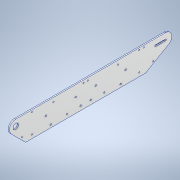
# Autodesk Inventor part: plyta_glowna_V3
Saved by Autodesk Inventor 2020.3 (Build 243373000, 373)
## iProperties
Created: 2021-04-10
Part Number: plyta_glowna_V3
Material: Aluminium 6061
Document SubType Name: Modeling
Designer: patryk.szydlik
Density: 2.7 g/cm^3
Appearance: Aluminium — płaski
Mass: 531.743 g
Surface Area: 1004.37 cm^2
Volume: 196.942 cm^3
Author: patryk.szydlik
Autodesk Inventor part; units mm, degrees
ref_plane "YZ Plane" through (0, 0, 0) normal (1, 0, 0) x (0, 1, 0)
ref_plane "XZ Plane" through (0, 0, 0) normal (0, 1, 0) x (-1, 0, 0)
ref_plane "XY Plane" through (0, 0, 0) normal (0, 0, 1) x (1, 0, 0)
sketch "Sketch2" plane through (0, 0, 0) normal (1, 0, 0) x (0, 1, 0)
  line L0 (127.2876, 96.9132) -> (-12.7124, 96.9132) construction
  line L1 (-12.7124, 96.9132) -> (-12.7124, -363.0868) construction
  line L2 (-12.7124, -363.0868) -> (127.2876, -363.0868) construction
  line L3 (127.2876, -363.0868) -> (127.2876, 96.9132) construction
  line L4 (97.2876, 66.9132) -> (17.2876, 66.9132) construction
  line L5 (17.2876, 66.9132) -> (17.2876, -333.0868) construction
  line L6 (17.2876, -333.0868) -> (97.2876, -333.0868) construction
  line L7 (97.2876, -333.0868) -> (97.2876, 66.9132) construction
  point P0 (0, 0)
  dimension "d2" = 140
  dimension "d3" = 460
  dimension "d4" = 80
  dimension "d5" = 400
  dimension "d6" = 30
  dimension "d7" = 30
  constraints: 16 end point, 4 parallel, 2 horizontal, 2 perpendicular
  measures "d2" distance of L2.end L1.end
  measures "d3" distance of L1.end L0.end
  measures "d4" distance of L6.end L5.end
  measures "d5" distance of L5.end L4.end
  measures "d6" distance between parallel lines of L3 L7
  measures "d7" distance between parallel lines of L0 L4
sketch "Sketch3" plane through (0, 0, 0) normal (1, 0, 0) x (0, 1, 0)
  circle A0 centre (-62.7124, 66.9132) radius 20
  line L0 (-12.7124, 96.9132) -> (-12.7124, -363.0868) construction
  circle A1 centre (-62.7124, -13.0868) radius 20
  circle A2 centre (-62.7124, -93.0868) radius 20
  circle A3 centre (-62.7124, -173.0868) radius 20
  circle A4 centre (-62.7124, -253.0868) radius 20
  circle A5 centre (-62.7124, -333.0868) radius 20
  line L1 (127.2876, 96.9132) -> (-12.7124, 96.9132) construction
  point P0 (0, 0)
  dimension "d8" = 40
  dimension "d9" = 50
  dimension "d12" = 80
  dimension "d17" = 30
  constraints: 6 centre point, 1 vertical, 10 other
  measures "d8" diameter of A0
  measures "d9" distance from line of L0 A0.centre
  measures "d12" distance of A0.centre A1.centre
  measures "d17" distance from line of A0.centre L1
sketch "Sketch1" plane through (0, 0, 0) normal (1, 0, 0) x (0, 1, 0)
  circle A0 centre (45.5719, 146.9132) radius 40
  circle A1 centre (85.5719, -453.0868) radius 40
  line L0 (127.2876, 96.9132) -> (-12.7124, 96.9132) construction
  line L1 (-12.7124, -363.0868) -> (127.2876, -363.0868) construction
  line L2 (-62.7124, 66.9132) -> (-62.7124, -13.0868) construction
  line L3 (-62.7124, -253.0868) -> (-62.7124, -333.0868) construction
  line L4 (85.2399, 141.7706) -> (125.4799, -450.3748) construction
  circle A2 centre (-62.7124, 66.9132) radius 20 projected
  line L5 (17.2876, 175.1975) -> (-76.8545, 81.0553)
  circle A3 centre (-62.7124, -333.0868) radius 20 projected
  line L6 (-76.8545, -347.2289) -> (57.2876, -481.3711) construction
  point P0 (0, 0)
  dimension "d0" = 80
  dimension "d1" = 80
  dimension "d18" = 50
  dimension "d19" = 90
  dimension "d45" = 135
  dimension "d46" = 135
  constraints: 10 end point, 4 point on circle, 3 tangent, 2 centre point, 2 coincident, 2 vertical, 6 other
  measures "d0" diameter of A0
  measures "d1" diameter of A1
  measures "d18" distance from line of A0.centre L0
  measures "d19" distance from line of A1.centre L1
  measures "d45" angle of L2 L5
  measures "d46" angle of L3 L6
sketch "Sketch4" plane through (0, 0, 0) normal (1, 0, 0) x (0, 1, 0)
  line L0 (37.6815, -3.0868) -> (-57.7124, 26.9132) construction
  circle A0 centre (-62.7124, 66.9132) radius 20 projected
  circle A1 centre (-62.7124, -13.0868) radius 20 projected
  line L1 (-62.7124, 66.9132) -> (-62.7124, -13.0868) construction
  circle A2 centre (-27.7124, 112.5679) radius 20 construction
  circle A3 centre (-27.7124, 32.5679) radius 20 construction
  line L2 (-27.7124, 72.5679) -> (37.6815, -3.0868) construction
  line L3 (-27.7124, 72.5679) -> (-57.7124, 26.9132) construction
  line L4 (37.6815, -3.0868) -> (-42.7124, 49.7406) construction
  line L5 (-12.7124, 96.9132) -> (-12.7124, -363.0868) construction
  point P0 (0, 0)
  point P1 (-61.7124, 47.9132)
  point P2 (83.0715, 79.9132)
  point P3 (83.0715, -80.0868)
  point P4 (37.6815, -163.0868)
  point P5 (83.0715, -240.0868)
  point P6 (37.6815, -323.0868)
  dimension "d22" = 40
  dimension "d23" = 5
  dimension "d24" = 30
  dimension "d25" = 40
  dimension "d26" = 40
  dimension "d27" = 80
  dimension "d28" = 40
  dimension "d29" = 100
  dimension "d30" = 100
  dimension "d31" = 35
  dimension "d32" = 54.6292
  dimension "d33" = 27.3146
  dimension "d34" = 56.691
  dimension "d35" = 95.3939
  dimension "d36" = 45.39
  dimension "d37" = 83
  dimension "d40" = 160
  constraints: 8 end point, 2 centre point, 2 vertical alignment, 1 coincident, 1 midpoint, 1 vertical, 4 other
  measures "d22" vertical distance of point (-62.712, 66.913) L0.end
  measures "d23" horizontal distance of point (-62.712, 66.913) L0.end
  measures "d24" vertical distance of L0.end L0.start
  measures "d25" diameter of A3
  measures "d26" diameter of A2
  measures "d27" distance of A3.centre A2.centre
  measures "d28" distance of A3.centre L2.start
  measures "d29" distance of L0.start L0.end
  measures "d30" distance of L2.start L0.start
  measures "d31" horizontal distance of point (-62.712, 66.913) A2.centre
  measures "d32" distance of L0.end L2.start
  measures "d33" distance of L0.end L4.end
  measures "d34" angle of L5 L4
  measures "d35" horizontal distance of L0.end L0.start
  measures "d36" horizontal distance of L0.start point (83.072, 79.913)
  measures "d37" vertical distance of L0.start point (83.072, 79.913)
  measures "d40" distance of point (83.072, 79.913) point (83.072, -80.087)
sketch "Sketch6" plane through (0, 0, 0) normal (1, 0, 0) x (0, 1, 0)
  line L0 (234.6261, -208.0868) -> (-157.479, -208.0868) construction
  line L1 (237.7494, -58.0868) -> (-154.3557, -58.0868) construction
  line L2 (17.2876, -333.0868) -> (97.2876, -333.0868) construction
  line L3 (97.2876, 66.9132) -> (17.2876, 66.9132) construction
  point P0 (0, 0)
  dimension "d61" = 125
  dimension "d62" = 125
  constraints: 4 end point, 2 horizontal
  measures "d61" distance between parallel lines of L1 L3
  measures "d62" distance between parallel lines of L2 L0
sketch "Sketch5" plane through (0, 0, 0) normal (1, 0, 0) x (0, 1, 0)
  arc A0 (90.5716, 146.9132) -> (47.894, 164.5909) centre (65.5716, 146.9132) ccw
  arc A1 (90.5716, -453.0868) -> (43.921, -465.5868) centre (65.5716, -453.0868) ccw construction
  line L0 (90.5716, -453.0868) -> (90.5716, 146.9132)
  arc A2 (47.894, 164.5909) -> (90.5716, 146.9132) centre (65.5716, 146.9132) ccw construction
  arc A3 (43.921, -465.5868) -> (90.5716, -453.0868) centre (65.5716, -453.0868) ccw
  arc A4 (62.5716, -453.0868) -> (68.5716, -453.0868) centre (65.5716, -453.0868) ccw
  arc A5 (68.5716, -413.0868) -> (62.5716, -413.0868) centre (65.5716, -413.0868) ccw
  line L1 (68.5716, -413.0868) -> (68.5716, -453.0868)
  line L2 (62.5716, -413.0868) -> (62.5716, -453.0868)
  arc A6 (68.5716, -453.0868) -> (62.5716, -453.0868) centre (65.5716, -453.0868) ccw construction
  arc A7 (62.5716, -413.0868) -> (68.5716, -413.0868) centre (65.5716, -413.0868) ccw construction
  line L3 (114.7874, 96.9132) -> (-25.2126, 96.9132) construction
  line L4 (-32.7126, -363.0868) -> (107.2874, -363.0868) construction
  line L5 (217.7491, -58.0868) -> (-174.356, -58.0868) construction
  line L6 (214.6258, -208.0868) -> (-177.4793, -208.0868) construction
  circle A8 centre (65.5716, 146.9132) radius 11
  circle A9 centre (65.5716, -413.0868) radius 50 construction
  circle A10 centre (65.5716, 146.9132) radius 55 construction
  line L7 (-9.4284, 107.2685) -> (47.894, 164.5909)
  line L8 (43.921, -465.5868) -> (-9.4284, -373.183)
  line L9 (-9.4284, -373.183) -> (-9.4284, 107.2685)
  line L10 (-2.7126, 66.9132) -> (-2.7126, -333.0868) construction
  line L11 (-62.7124, -13.0868) -> (-62.7124, -93.0868) construction
  line L12 (-62.7124, -173.0868) -> (-62.7124, -253.0868) construction
  point P0 (0, 0)
  point P1 (83.0716, 81.9132)
  point P2 (83.0716, -348.0868)
  point P3 (83.0716, -366.2493)
  point P4 (16.3276, 122.4179)
  point P5 (5.5716, -347.5476)
  point P6 (16.5597, -403.1957)
  point P7 (8.0719, -82.4742)
  point P8 (8.0719, -243.0868)
  point P9 (-17.7126, -58.0868)
  point P10 (-17.7126, -208.0868)
  point P11 (5.5716, 81.9132)
  point P12 (-62.7124, 66.9132)
  point P13 (-62.7124, -333.0868)
  point P14 (-62.7124, -53.0868)
  point P15 (-62.7124, -213.0868)
  point P16 (2.2876, 6.9132)
  point P17 (42.2876, 26.9132)
  point P18 (47.2876, -93.0868)
  point P19 (7.2876, -113.0868)
  point P20 (7.2876, -153.0868)
  point P21 (47.2876, -173.0868)
  point P22 (42.2876, -293.0868)
  point P23 (2.2876, -273.0868)
  point P24 (2.2876, 6.9132)
  point P25 (-62.7124, 66.9132)
  point P26 (5.5716, -208.0868)
  point P27 (5.5716, -58.0868)
  point P28 (75.1946, -4.4068)
  point P29 (80.1946, -124.4068)
  point P30 (80.1946, -141.7668)
  point P31 (75.1946, -261.7668)
  dimension "d84" = 110
  dimension "d47" = 50
  dimension "d48" = 50
  dimension "d58" = 6
  dimension "d59" = 6
  dimension "d60" = 40
  dimension "d63" = 15
  dimension "d64" = 7.5
  dimension "d65" = 15
  dimension "d66" = 7.5
  dimension "d81" = 22
  dimension "d82" = 100
  dimension "d86" = 100
  dimension "d92" = 7.5
  dimension "d101" = 7.5
  dimension "d102" = 7.5
  dimension "d103" = 135
  dimension "d104" = 150
  dimension "d151" = 15
  dimension "d155" = 15
  dimension "d159" = 15
  dimension "d160" = 15
  dimension "d163" = 60
  dimension "d164" = 65
  dimension "d165" = 20
  dimension "d166" = 40
  dimension "d174" = 60
  dimension "d175" = 70
  dimension "d176" = 40
  dimension "d177" = 20
  dimension "d196" = 128.284
  dimension "d197" = 15
  dimension "d198" = 11.32
  dimension "d199" = 72.907
  dimension "d200" = 11.32
  dimension "d201" = 72.907
  dimension "d204" = 11.32
  dimension "d213" = 65
  dimension "d214" = 40
  dimension "d215" = 20
  dimension "d216" = 20
  dimension "d217" = 40
  constraints: 26 end point, 18 point on circle, 10 centre point, 8 coincident, 4 point on line, 2 midpoint, 1 vertical alignment, 3 other
  measures "d47" diameter of A0
  measures "d48" diameter of A1
  measures "d58" diameter of A4
  measures "d59" diameter of A5
  measures "d60" distance of point (65.572, -453.087) point (65.572, -413.087)
  measures "d63" distance from line of L3 point (83.072, 81.913)
  measures "d64" distance from line of L0 point (83.072, 81.913)
  measures "d65" distance from line of L4 point (83.072, -348.087)
  measures "d66" distance from line of L0 point (83.072, -348.087)
  measures "d81" diameter of A8
  measures "d82" diameter of A9
  measures "d86" distance between parallel lines of L9 L0
  measures "d92" distance from line of L0 A9.start
  measures "d101" distance from line of point (16.328, 122.418) L7
  measures "d102" distance from line of L8 A9.end
  measures "d103" angle of L7 L9
  measures "d104" angle of L9 L8
  measures "d151" distance from line of L10 point (-17.713, -58.087)
  measures "d155" distance from line of L10 point (-17.713, -208.087)
  measures "d159" distance from line of L3 point (5.572, 81.913)
  measures "d160" distance from line of L9 point (5.572, 81.913)
  measures "d163" vertical distance of point (-62.712, 66.913) point (2.288, 6.913)
  measures "d164" horizontal distance of point (-62.712, 66.913) point (2.288, 6.913)
  measures "d165" vertical distance of point (2.288, 6.913) point (42.288, 26.913)
  measures "d166" horizontal distance of point (2.288, 6.913) point (42.288, 26.913)
  measures "d174" vertical distance of point (-62.712, -213.087) point (7.288, -153.087)
  measures "d175" horizontal distance of point (-62.712, -213.087) point (7.288, -153.087)
  measures "d176" horizontal distance of point (47.288, -173.087) point (7.288, -153.087)
  measures "d177" vertical distance of point (47.288, -173.087) point (7.288, -153.087)
  measures "d196" horizontal distance of point (65.572, 146.913) point (-62.712, 66.913)
  measures "d197" distance from line of point (5.572, -347.548) L9
  measures "d198" vertical distance of point (75.195, -4.407) point (2.288, 6.913)
  measures "d199" horizontal distance of point (2.288, 6.913) point (75.195, -4.407)
  measures "d200" vertical distance of point (7.288, -113.087) point (80.195, -124.407)
  measures "d201" horizontal distance of point (7.288, -113.087) point (80.195, -124.407)
  measures "d204" vertical distance of point (2.288, -273.087) point (75.195, -261.767)
  measures "d213" horizontal distance of point (2.288, -273.087) L12.end
  measures "d214" horizontal distance of point (2.288, -273.087) point (42.288, -293.087)
  measures "d215" vertical distance of point (2.288, -273.087) point (42.288, -293.087)
  measures "d216" vertical distance of point (7.288, -113.087) point (47.288, -93.087)
  measures "d217" horizontal distance of point (47.288, -93.087) point (7.288, -113.087)
extrude "Extrusion1" add sketch "Sketch5" against normal blind 5
hole "Hole1" at (0, 83.0716, 81.9132) at (0, 16.3276, 122.4179) at (0, 5.5716, -347.5476) at (0, 16.5597, -403.1957) at (0, 83.0716, -348.0868) at (0, 83.0716, -366.2493) at (0, -17.7126, -58.0868) at (0, -17.7126, -208.0868) at (0, 5.5716, 81.9132) at (0, 5.5716, -58.0868) at (0, 5.5716, -208.0868) direction (-1, 0, 0) diameter 5 end through all clearance for "Flat Head Machine Screw" size "M5" standard "Ansi Metric M Profile"
sketch "Sketch7" plane through (0, 0, 0) normal (1, 0, 0) x (0, 0, -1)
  circle A0 centre (348.0868, 83.0716) radius 2.5 projected
  circle A1 centre (-122.4179, 16.3276) radius 2.5 projected
  circle A2 centre (-81.9132, 83.0716) radius 2.5 projected
  circle A3 centre (403.1957, 16.5597) radius 2.5 projected
  circle A4 centre (366.2493, 83.0716) radius 2.5 projected
  line L0 (373.183, -9.4284) -> (465.5868, 43.921) projected
  arc A5 (465.5868, 43.921) -> (453.0868, 90.5716) centre (453.0868, 65.5716) ccw projected
  line L1 (453.0868, 90.5716) -> (-146.9132, 90.5716) projected
  arc A6 (-146.9132, 90.5716) -> (-164.5909, 47.894) centre (-146.9132, 65.5716) ccw projected
  line L2 (-164.5909, 47.894) -> (-107.2685, -9.4284) projected
  circle A7 centre (-146.9132, 65.5716) radius 11 projected
  arc A8 (453.0868, 62.5716) -> (453.0868, 68.5716) centre (453.0868, 65.5716) ccw projected
  line L3 (453.0868, 62.5716) -> (413.0868, 62.5716) projected
  arc A9 (413.0868, 68.5716) -> (413.0868, 62.5716) centre (413.0868, 65.5716) ccw projected
  line L4 (413.0868, 68.5716) -> (453.0868, 68.5716) projected
  line L5 (-146.9132, 75.5716) -> (453.0868, 75.5716)
  arc A10 (458.0868, 56.9114) -> (453.0868, 75.5716) centre (453.0868, 65.5716) ccw
  line L6 (458.0868, 56.9114) -> (386.4847, 15.5719)
  line L7 (386.4847, 15.5719) -> (398.0868, 15.5719)
  line L8 (-111.0556, 15.5719) -> (-153.9843, 58.5006)
  arc A11 (-146.9132, 75.5716) -> (-153.9843, 58.5006) centre (-146.9132, 65.5716) ccw
  line L9 (453.0868, 90.5716) -> (-146.9132, 90.5716) projected
  line L10 (-91.9132, 90.5716) -> (-71.9132, 90.5716)
  line L11 (-71.9132, 90.5716) -> (-71.9132, 0.5716)
  line L12 (-71.9132, 0.5716) -> (-91.9132, 0.5716)
  line L13 (-91.9132, 0.5716) -> (-91.9132, 90.5716)
  line L14 (-107.2685, -9.4284) -> (373.183, -9.4284) projected
  line L15 (48.0868, 90.5716) -> (68.0868, 90.5716)
  line L16 (68.0868, 90.5716) -> (68.0868, -9.4284)
  line L17 (68.0868, -9.4284) -> (48.0868, -9.4284)
  line L18 (48.0868, -9.4284) -> (48.0868, 90.5716)
  line L19 (198.0868, 90.5716) -> (218.0868, 90.5716)
  line L20 (218.0868, 90.5716) -> (218.0868, -9.4284)
  line L21 (218.0868, -9.4284) -> (198.0868, -9.4284)
  line L22 (198.0868, -9.4284) -> (198.0868, 90.5716)
  line L23 (338.0868, 90.5716) -> (358.0868, 90.5716)
  line L24 (358.0868, 90.5716) -> (358.0868, 38.7433)
  line L25 (358.0868, -9.4284) -> (338.0868, -9.4284)
  line L26 (338.0868, -9.4284) -> (338.0868, 90.5716)
  circle A12 centre (-146.9132, 65.5719) radius 25 construction
  arc A13 (453.0868, 62.5716) -> (453.0868, 68.5716) centre (453.0868, 65.5716) ccw construction
  circle A14 centre (453.0868, 65.5716) radius 25 construction
  arc A15 (413.0868, 68.5716) -> (413.0868, 62.5716) centre (413.0868, 65.5716) ccw construction
  line L27 (-146.9132, 90.5716) -> (453.0868, 90.5716) construction
  line L28 (398.0911, 65.9311) -> (398.0911, 90.5716) construction
  line L29 (403.0868, 38.7433) -> (456.6188, 38.7433) construction
  line L30 (465.5868, 43.921) -> (373.183, -9.4284) construction
  line L31 (403.0868, 38.7433) -> (403.0868, 15.5719) construction
  line L32 (398.0868, 65.5716) -> (398.0868, 38.7433) construction
  line L33 (398.0868, 38.7433) -> (398.0868, 38.7433) construction
  line L34 (398.0868, 15.5719) -> (398.0868, 38.7433) construction
  line L35 (408.0868, 38.7433) -> (408.0868, 15.5716) construction
  line L36 (358.0868, 38.7433) -> (358.0868, -9.4284)
  line L37 (398.0868, 38.7433) -> (403.0868, 38.7433) construction
  line L38 (398.0868, 15.5719) -> (-111.0556, 15.5719)
  line L39 (218.0868, 75.5716) -> (338.0868, 15.5719) construction
  line L40 (218.0868, 15.5719) -> (338.0868, 75.5716) construction
  line L41 (326.9064, 75.5716) -> (218.0868, 21.1621) construction
  line L42 (229.2672, 15.5719) -> (338.0868, 69.9815) construction
  line L43 (229.2672, 75.5716) -> (338.0868, 21.1621) construction
  line L44 (218.0868, 69.9815) -> (326.9064, 15.5719) construction
  line L45 (333.0869, 67.4815) -> (333.0869, 23.662) construction
  line L46 (68.0868, 75.5716) -> (198.0868, 15.5719) construction
  line L47 (198.0868, 75.5716) -> (68.0868, 15.5719) construction
  line L48 (68.0868, 21.0787) -> (186.1552, 75.5716) construction
  line L49 (80.0184, 15.5719) -> (198.0868, 70.0648) construction
  line L50 (198.0868, 21.0787) -> (80.0184, 75.5716) construction
  line L51 (68.0868, 70.0648) -> (186.1552, 15.5719) construction
  line L52 (48.0868, 15.5719) -> (-71.9132, 75.5716) construction
  line L53 (-71.9132, 15.5719) -> (48.0868, 75.5716) construction
  line L54 (36.9064, 75.5716) -> (-71.9132, 21.1621) construction
  line L55 (-60.7328, 15.5719) -> (48.0868, 69.9815) construction
  line L56 (-60.7328, 75.5716) -> (48.0868, 21.1621) construction
  line L57 (-71.9132, 69.9815) -> (36.9064, 15.5719) construction
  line L58 (68.0868, 73.0713) -> (61.5727, 73.0713) construction
  line L59 (48.0868, 47.6814) -> (-4.9521, 47.6814) construction
  line L60 (198.0868, 47.6814) -> (140.4475, 47.6814) construction
  line L61 (218.0868, 73.0713) -> (211.9072, 73.0713) construction
  line L62 (-121.9132, 65.5719) -> (-121.9132, 75.5716) construction
  line L63 (-121.9132, 65.5719) -> (-121.9132, 26.4295) construction
  line L64 (-121.9132, 75.5716) -> (-91.9132, 15.5719) construction
  line L65 (-91.9132, 26.7522) -> (-116.323, 75.5716) construction
  line L66 (-121.9132, 64.3913) -> (-97.5034, 15.5719) construction
  line L67 (-111.0556, 15.5719) -> (-121.9132, 15.5719) construction
  line L68 (-121.9132, 15.5719) -> (-121.9132, 26.4295) construction
  line L69 (-121.9132, 15.5719) -> (-91.9132, 75.5716) construction
  line L70 (-97.5034, 75.5716) -> (-121.9132, 26.7522) construction
  line L71 (-116.323, 15.5719) -> (-91.9132, 64.3913) construction
  circle A16 centre (413.0868, 65.5716) radius 15 construction
  line L72 (398.0911, 75.5716) -> (358.0868, 15.5719) construction
  line L73 (398.0868, 15.5719) -> (358.0868, 75.5716) construction
  line L74 (392.0816, 75.5716) -> (358.0868, 24.5851) construction
  line L75 (398.0911, 66.5584) -> (364.0963, 15.5719) construction
  line L76 (358.0868, 66.5578) -> (392.0775, 15.5719) construction
  line L77 (398.0868, 24.5857) -> (364.0961, 75.5716) construction
  line L78 (-107.2685, -9.4284) -> (373.183, -9.4284) projected
  point P0 (0, 0)
  dimension "d93" = 15
  dimension "d94" = 10
  dimension "d95" = 20
  dimension "d97" = 20
  dimension "d99" = 20
  dimension "d100" = 10
  dimension "d105" = 20
  dimension "d107" = 5
  dimension "d108" = 5
  dimension "d111" = 5
  dimension "d112" = 5
  dimension "d113" = 5
  dimension "d114" = 5
  dimension "d116" = 5
  dimension "d117" = 5
  dimension "d118" = 5
  dimension "d119" = 5
  dimension "d120" = 5
  dimension "d121" = 5
  dimension "d122" = 5
  dimension "d123" = 5
  dimension "d128" = 5
  dimension "d129" = 5
  dimension "d130" = 5
  dimension "d131" = 5
  dimension "d132" = 30
  dimension "d133" = 5
  dimension "d134" = 5
  dimension "d135" = 5
  dimension "d136" = 5
  constraints: 134 end point, 57 point on line, 29 parallel, 11 perpendicular, 9 horizontal, 6 point on circle, 6 vertical, 4 centre point, 3 coincident, 1 collinear, 1 concentric, 1 horizontal alignment, 1 vertical alignment, 54 other
  measures "d94" distance from line of L11 A2.centre
  measures "d95" distance of L16.end L17.end
  measures "d97" distance of L20.end L21.end
  measures "d99" distance of L25.start L25.end
  measures "d100" distance from line of L24 A0.centre
  measures "d105" distance between parallel lines of L11 L13
  measures "d107" distance between parallel lines of L34 L31
  measures "d108" distance between parallel lines of L31 L35
  measures "d111" distance between parallel lines of L41 L40
  measures "d112" distance between parallel lines of L40 L42
  measures "d113" distance between parallel lines of L39 L43
  measures "d114" distance between parallel lines of L44 L39
  measures "d116" distance between parallel lines of L49 L47
  measures "d117" distance between parallel lines of L48 L47
  measures "d118" distance between parallel lines of L50 L46
  measures "d119" distance between parallel lines of L51 L46
  measures "d120" distance between parallel lines of L56 L52
  measures "d121" distance between parallel lines of L57 L52
  measures "d122" distance between parallel lines of L53 L54
  measures "d123" distance between parallel lines of L55 L53
  measures "d128" distance between parallel lines of L64 L65
  measures "d129" distance between parallel lines of L64 L66
  measures "d130" distance between parallel lines of L71 L69
  measures "d131" distance between parallel lines of L70 L69
  measures "d132" diameter of A16
  measures "d133" distance between parallel lines of L72 L74
  measures "d134" distance between parallel lines of L75 L72
  measures "d135" distance between parallel lines of L77 L73
  measures "d136" distance between parallel lines of L76 L73
hole "Otwór2" at (0, 2.2876, 6.9132) at (0, 42.2876, 26.9132) at (0, 7.2876, -113.0868) at (0, 47.2876, -93.0868) at (0, 7.2876, -153.0868) at (0, 47.2876, -173.0868) at (0, 2.2876, -273.0868) at (0, 42.2876, -293.0868) direction (-1, 0, 0) diameter 6 end through all
hole "Otwór3" at (0, 75.1946, -4.4068) at (0, 80.1946, -141.7668) at (0, 80.1946, -124.4068) at (0, 75.1946, -261.7668) direction (-1, 0, 0) diameter 5 end through all
equation "\"d28\" = 0.5 * d27"
equation "\"d30\" = d29"
equation "\"d33\" = 0.5 * d32"
equation "\"d62\" = d61"
body "Solid1"
